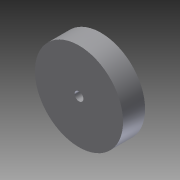
# Autodesk Inventor part: gearMountSpacer
Saved by Autodesk Inventor 2012 (Build 160160000, 160)
## iProperties
Created: 2014-06-12
Part Number: gearMountSpacer
Material: Default
Document SubType Name: Modeling
Designer: Byron
Density: 1 g/cm^3
Author: Byron
Autodesk Inventor part; units mm, degrees
ref_plane "YZ Plane" through (0, 0, 0) normal (1, 0, 0) x (0, 1, 0)
ref_plane "XZ Plane" through (0, 0, 0) normal (0, 1, 0) x (-1, 0, 0)
ref_plane "XY Plane" through (0, 0, 0) normal (0, 0, 1) x (1, 0, 0)
sketch "Sketch1" plane through (0, 0, 0) normal (0, 0, 1) x (1, 0, 0)
  circle A0 centre (31.416, 0) radius 3.175 projected
  arc A1 (56.214, 44.45) -> (49.864, 50.8) centre (49.864, 44.45) ccw projected
  line L0 (-49.864, 50.8) -> (49.864, 50.8) projected
  arc A2 (-49.864, 50.8) -> (-56.214, 44.45) centre (-49.864, 44.45) ccw projected
  line L1 (-56.214, -44.45) -> (-56.214, 44.45) projected
  arc A3 (-56.214, -44.45) -> (-49.864, -50.8) centre (-49.864, -44.45) ccw projected
  line L2 (49.864, -50.8) -> (-49.864, -50.8) projected
  arc A4 (49.864, -50.8) -> (56.214, -44.45) centre (49.864, -44.45) ccw projected
  line L3 (56.214, 44.45) -> (56.214, -44.45) projected
  circle A5 centre (-24.464, 35.97) radius 12.7
  circle A6 centre (-11.2704, 9.7076) radius 3.175 projected
  circle A7 centre (12.9836, 43.4062) radius 3.175 projected
  circle A8 centre (-24.464, 35.97) radius 3.175 projected
  circle A9 centre (9.7431, -32.1205) radius 2.5 projected
  point P0 (0, 0)
  dimension "d0" = 25.4
  constraints: 1 centre point
  measures "d0" diameter of A5
extrude "Extrusion1" add sketch "Sketch1" along normal blind 6.35 contours A5 | A8
body "Solid1"
